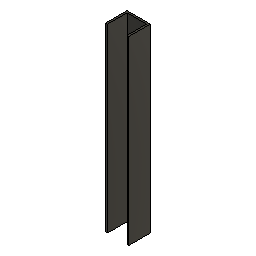
2020 Shelf Bracket Spacer v7 (Autodesk Fusion 360 design; units mm, degrees)
Autodesk Fusion 360 part; units mm, degrees
sketch "Sketch1" plane through (0, 0, 0) normal (0, 0, 1) x (1, 0, 0) in component "Spacer"
  line L0 (0, 0) -> (20, 0)
  line L1 (20, 0) -> (20, 20)
  line L2 (20, 20) -> (0, 20)
  line L3 (0, 20) -> (0, 0)
  line L4 (-0.2, -0.2) -> (20.2, -0.2)
  line L5 (20.2, -0.2) -> (20.2, 20.2)
  line L6 (20.2, 20.2) -> (-0.2, 20.2)
  line L7 (-0.2, 20.2) -> (-0.2, -0.2)
  line L8 (-0.2, -0.2) -> (-2.2, -0.2)
  line L9 (-2.2, -0.2) -> (-2.2, 22.2)
  line L10 (-2.2, 22.2) -> (22.2, 22.2)
  line L11 (22.2, 22.2) -> (22.2, -0.2)
  line L12 (22.2, -0.2) -> (20.2, -0.2)
  dimension "d1" = 20
  dimension "d2" = 20
  dimension "d3" = 0.2
  dimension "d4" = 2
  dimension "d5" = 22.4
  dimension "d6" = 2
  dimension "d7" = 22.4
  dimension "d8" = 24.4
  constraint horizontal L0
  constraint vertical L1
  constraint horizontal L2
  constraint vertical L3
  constraint coincident L0.start L3.end
  constraint perpendicular L7 L8
  constraint perpendicular L4 L9
  constraint perpendicular L9 L10
  measures "d1" distance of L0.start L2.end
  measures "d2" distance of L0.start L0.end
  measures "d4" distance of L4.start L8.end
  measures "d5" distance of L8.end L9.end
  measures "d6" horizontal distance of L4.end L11.end
  measures "d7" vertical distance of L10.end L11.end
  measures "d8" distance of L9.end L10.end
extrude "Extrude1" add sketch "Sketch1" along normal blind 189.5 contours L5 L6 L7 L8 L9 L10 L11 L12 in component "Spacer"
sketch "Sketch1 (2)" plane through (0, 20.2, 0) normal (0, -1, 0) x (1, 0, 0)
  line L0 (-0.2, 0) -> (20.2, 0)
  line L1 (20.2, 0) -> (20.2, 189.5)
  line L2 (20.2, 189.5) -> (-0.2, 189.5)
  line L3 (-0.2, 189.5) -> (-0.2, 0)
  line L4 (15.4697, 11.1014) -> (15.4697, 184.8015) construction
  line L5 (15.4697, 184.8015) -> (5.7417, 184.8015) construction
  line L6 (5.7417, 184.8015) -> (5.7417, 11.1014) construction
  line L7 (5.7417, 11.1014) -> (15.4697, 11.1014) construction
  dimension "d14" = 8
  dimension "d15" = 0
  text T0 "189.5 mm v7" font "Arial" height 8 align centre middle in box 173.7001 x 9.728 at (15.4697, 11.1014) x (0, 1) y (-1, 0) spacing 1
emboss "Emboss1" depth -1 profiles "Sketch1 (2)" section 1 text T0 onto face at (13.4, 20.2, 63.1667) in component "Spacer"
component "Spacer" placed x (1, 0, 0) y (0, 1, 0) z (0, 0, 1) at (0, 0, 0)
equation "d9 = Length"
equation "Length = 189.5 mm"
equation "LengthText = Length"
equation "d15 = LengthText + ' ' + PublishedVersion"
equation "PublishedVersion = 'v7'"
